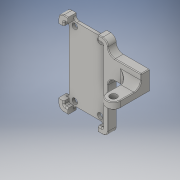
# Autodesk Inventor part: Wall Mount
Saved by Autodesk Inventor 2016 (Build 200138000, 138)
## iProperties
Created: 2019-03-14
Part Number: Wall Mount
Material: Generic
Document SubType Name: Modeling
Designer: HAL-9000
Density: 1 g/cm^3
Appearance: Default
Author: HAL-9000
Autodesk Inventor part; units mm, degrees
note: some values were not read from the file. Chosen so that the rebuilt part matches the saved one: sketch regions of "Extrusion1".
ref_plane "YZ Plane" through (0, 0, 0) normal (1, 0, 0) x (0, 1, 0)
ref_plane "XZ Plane" through (0, 0, 0) normal (0, 1, 0) x (-1, 0, 0)
ref_plane "XY Plane" through (0, 0, 0) normal (0, 0, 1) x (1, 0, 0)
sketch "Sketch1" plane through (0, 0, 0) normal (0, 0, 1) x (1, 0, 0)
  line L0 (0, 0) -> (35.56, 0)
  line L1 (35.56, 0) -> (35.56, 67.31)
  line L2 (35.56, 67.31) -> (0, 67.31)
  line L3 (0, 67.31) -> (0, 0)
  line L4 (-5.08, 3.81) -> (-5.08, 0)
  line L5 (3.81, -5.08) -> (0, -5.08)
  arc A0 (-5.08, 0) -> (0, -5.08) centre (0, 0) ccw
  line L6 (-5.08, 3.81) -> (0, 3.81)
  line L7 (3.81, -5.08) -> (3.81, 0)
  line L8 (3.81, 0) -> (0, 0)
  line L9 (0, 0) -> (0, 3.81)
  line L10 (17.78, 67.31) -> (17.78, 0)
  line L11 (0, 33.655) -> (35.56, 33.655)
  line L12 (-5.08, 63.5) -> (-5.08, 67.31)
  line L13 (3.81, 72.39) -> (0, 72.39)
  arc A1 (0, 72.39) -> (-5.08, 67.31) centre (0, 67.31) ccw
  line L14 (-5.08, 63.5) -> (0, 63.5)
  line L15 (3.81, 72.39) -> (3.81, 67.31)
  line L16 (3.81, 67.31) -> (0, 67.31)
  line L17 (0, 67.31) -> (0, 63.5)
  line L18 (40.64, 3.81) -> (40.64, 0)
  line L19 (31.75, -5.08) -> (35.56, -5.08)
  arc A2 (35.56, -5.08) -> (40.64, 0) centre (35.56, 0) ccw
  line L20 (40.64, 3.81) -> (35.56, 3.81)
  line L21 (31.75, -5.08) -> (31.75, 0)
  line L22 (31.75, 0) -> (35.56, 0)
  line L23 (35.56, 0) -> (35.56, 3.81)
  line L24 (40.64, 63.5) -> (35.56, 63.5)
  line L25 (40.64, 63.5) -> (40.64, 67.31)
  line L26 (35.56, 67.31) -> (35.56, 63.5)
  line L27 (31.75, 67.31) -> (35.56, 67.31)
  line L28 (31.75, 72.39) -> (31.75, 67.31)
  line L29 (31.75, 72.39) -> (35.56, 72.39)
  arc A3 (40.64, 67.31) -> (35.56, 72.39) centre (35.56, 67.31) ccw
  circle A4 centre (28.448, 63.5) radius 2.54
  circle A5 centre (28.448, 3.81) radius 2.54
  circle A6 centre (5.08, 3.81) radius 2.54
  circle A7 centre (5.08, 63.5) radius 2.54
  line L30 (35.56, 63.5) -> (40.64, 63.5)
  line L31 (40.64, 63.5) -> (40.64, 3.81)
  line L32 (40.64, 3.81) -> (35.56, 3.81)
  line L33 (35.56, 3.81) -> (35.56, 63.5)
  point P0 (35.56, 0)
  point P1 (35.56, 67.31)
  dimension "d0" = 67.31
  dimension "d1" = 35.56
  dimension "d2" = 5.08
  dimension "d3" = 5.08
  dimension "d4" = 0
  dimension "d5" = 0
  dimension "d6" = 3.81
  dimension "d7" = 3.81
  dimension "d8" = 17.78
  dimension "d9" = 33.655
  dimension "d10" = 1.27
  dimension "d11" = 4.572
  dimension "d12" = 5.08
  dimension "d13" = 5.08
  dimension "d14" = 1.27
  dimension "d15" = 2.54
  constraints: 68 end point, 26 symmetric about line, 8 centre point, 8 point on circle, 6 parallel, 6 perpendicular, 4 midpoint, 3 horizontal, 2 point on line, 1 tangent, 5 other
  measures "d0" distance between parallel lines of L0 L2
  measures "d1" distance between parallel lines of L1 L3
  measures "d2" distance between parallel lines of L3 L4
  measures "d3" distance between parallel lines of L5 L0
  measures "d4" vertical distance of L0.start L4.end
  measures "d5" horizontal distance of L0.start L5.end
  measures "d6" distance from line of L0 L4.start
  measures "d7" distance from line of L5.start L3
  measures "d8" distance between parallel lines of L3 L10
  measures "d9" distance between parallel lines of L0 L11
  measures "d10" distance edge to line of A4 L2
  measures "d11" distance edge to line of A4 L1
  measures "d12" diameter of A4
  measures "d13" diameter of A6
  measures "d14" distance edge to line of A6 L0
  measures "d15" distance edge to line of A6 L3
extrude "Extrusion1" add sketch "Sketch1" along normal blind 2.54
extrude "Extrusion2" add sketch "Sketch1" along normal blind 7.62 contours L0 L7 L5 A0 L4 L6 L3 | L0 L1 L20 L18 A2 L19 L21 | L14 L12 A1 L13 L15 L2 L3 | L1 L24 L31 L20 | L28 L29 A3 L25 L24 L1 L2
fillet "Fillet1" radius 3.175 6 edges at (3.81, 67.31, 1.27) (31.75, 67.31, 1.27) (3.81, 0, 1.27) (31.75, 0, 1.27) (0, 3.81, 1.27) (0, 63.5, 1.27)
fillet "Fillet2" radius 1.27 4 edges at (0, 67.31, 5.08) (35.56, 67.31, 5.08) (0, 0, 5.08) (35.56, 0, 5.08)
fillet "Fillet3" radius 1.27 11 edges at (0.372, 0.372, 7.62) (2.54, 0, 7.62) (0, 2.54, 7.62) (35.56, 33.655, 7.62) (35.188, 66.938, 7.62) (33.02, 67.31, 7.62) (33.02, 0, 7.62) (35.188, 0.372, 7.62) (0.372, 66.938, 7.62) (2.54, 67.31, 7.62) (0, 64.77, 7.62)
sketch "Sketch2" plane through (0, 0, 0) normal (0, 0, -1) x (-1, 0, 0)
  line L0 (-40.64, 0) -> (-40.64, 67.31) projected
  line L1 (-40.64, 60.96) -> (-71.12, 60.96)
  line L2 (-71.12, 60.96) -> (-71.12, 43.18)
  line L3 (-71.12, 43.18) -> (-40.64, 43.18)
  line L4 (-40.64, 43.18) -> (-40.64, 60.96)
  point P0 (0, 0)
  dimension "d23" = 17.78
  dimension "d24" = 6.35
  dimension "d25" = 30.48
  constraints: 8 end point, 2 parallel, 1 horizontal, 1 perpendicular, 1 point on line
  measures "d23" distance between parallel lines of L3 L1
  measures "d24" distance from line of L0.end L1
  measures "d25" distance between parallel lines of L0 L2
extrude "Extrusion3" add sketch "Sketch2" against normal up to surface (7.62 mm away)
fillet "Fillet4" radius 6.35 2 edges at (40.64, 60.96, 3.81) (40.64, 43.18, 3.81)
sketch "Sketch3" plane through (71.12, 43.18, 0) normal (1, 0, 0) x (0, 0, -1)
  line L0 (-7.62, 0) -> (-7.62, -6.35) projected
  line L1 (-7.62, 0) -> (-33.02, 0)
  line L2 (-33.02, 0) -> (-33.02, 6.35)
  line L3 (-33.02, 6.35) -> (-7.62, 6.35)
  line L4 (-7.62, 6.35) -> (-7.62, 0)
  point P0 (0, -43.18)
  dimension "d29" = 6.35
  dimension "d30" = 25.4
  constraints: 8 end point, 2 parallel, 1 horizontal, 1 perpendicular
  measures "d29" distance between parallel lines of L1 L3
  measures "d30" distance between parallel lines of L4 L2
extrude "Extrusion4" add sketch "Sketch3" against normal blind 12.7
fillet "Fillet5" radius 6.35 4 edges at (64.77, 49.53, 7.62) (58.42, 46.355, 7.62) (71.12, 46.355, 33.02) (58.42, 46.355, 33.02)
sketch "Sketch4" plane through (71.12, 49.53, 26.67) normal (0, 1, 0) x (1, 0, 0)
  circle A0 centre (-6.35, 0) radius 3.175
  arc A1 (-12.7, 0) -> (0, 0) centre (-6.35, 0) ccw projected
  point P0 (-71.12, 26.67)
  dimension "d34" = 6.35
  constraints: 1 centre point, 1 concentric
  measures "d34" diameter of A0
extrude "Extrusion5" cut sketch "Sketch4" against normal blind 12.7
fillet "Fillet6" radius 0.635 26 edges at (58.42, 49.53, 20.32) (56.5602, 51.3898, 9.4798) (71.12, 49.53, 20.32) (71.12, 51.3898, 9.4798) (71.12, 58.42, 7.62) (69.2602, 49.53, 31.1602) (71.12, 43.18, 13.3351) (58.42, 43.18, 20.32) (56.5602, 43.18, 9.4798) (49.53, 43.18, 7.62) (42.4998, 41.3202, 7.62) (40.64, 18.4151, 7.62) (39.1521, -3.5921, 7.62) (33.655, -5.08, 7.62) (69.2602, 43.18, 31.1602) (40.64, 67.31, 7.62) (39.1521, 70.9021, 7.62) (33.655, 72.39, 7.62) (59.0549, 60.96, 7.62) (71.12, 60.96, 3.81) (1.905, -5.08, 7.62) (-5.08, 1.905, 7.62) (-3.5921, -3.5921, 7.62) (-5.08, 65.405, 7.62) (1.905, 72.39, 7.62) (-3.5921, 70.9021, 7.62)
body "Solid1"
